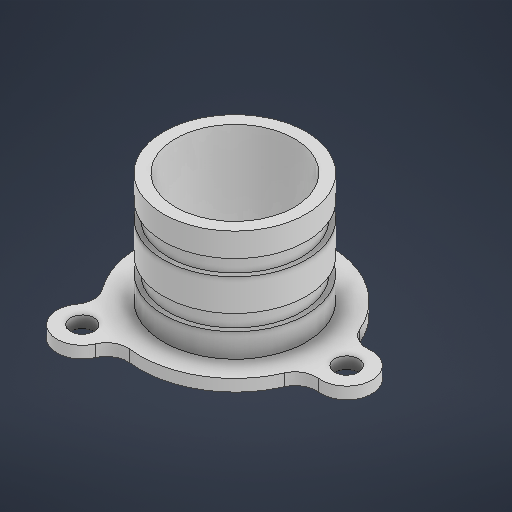
# Autodesk Inventor part: 10
Saved by Autodesk Inventor 2025.4 (Build 294407000, 407)
## iProperties
Created: 2026-05-07
Part Number: 10
Material: Generic
Document SubType Name: Modeling
Designer: VuQuan
Density: 1 g/cm^3
Appearance: Default
Author: VuQuan
Autodesk Inventor part; units mm, degrees
ref_plane "YZ Plane" through (0, 0, 0) normal (1, 0, 0) x (0, 1, 0)
ref_plane "XZ Plane" through (0, 0, 0) normal (0, 1, 0) x (-1, 0, 0)
ref_plane "XY Plane" through (0, 0, 0) normal (0, 0, 1) x (1, 0, 0)
sketch "Sketch1" plane through (0, 0, 0) normal (0, 0, 1) x (1, 0, 0)
  line L0 (0, 0) -> (0, 77.5) construction
  line L1 (45, 77.5) -> (45, 62.5)
  line L2 (45, 62.5) -> (42, 62.5)
  line L3 (42, 62.5) -> (42, 52.5)
  line L4 (42, 52.5) -> (45, 52.5)
  line L5 (45, 52.5) -> (45, 32.5)
  line L6 (45, 32.5) -> (42, 32.5)
  line L7 (42, 32.5) -> (42, 22.5)
  line L8 (42, 22.5) -> (45, 22.5)
  line L9 (45, 22.5) -> (45, 7.5)
  line L10 (45, 77.5) -> (37.5, 77.5)
  line L11 (37.5, 77.5) -> (37.5, 7.5)
  line L12 (37.5, 7.5) -> (45, 7.5)
  dimension "d0" = 3
  dimension "d1" = 15
  dimension "d2" = 10
  dimension "d3" = 20
  dimension "d4" = 7.5
  dimension "d5" = 15
  dimension "d6" = 90
  dimension "d7" = 77.5
  dimension "d8" = 75
  constraints: 26 end point, 8 perpendicular, 3 point on line, 2 collinear, 2 horizontal, 2 vertical
  measures "d0" distance of L7.end L8.end
  measures "d1" distance of L1.start L1.end
  measures "d2" distance of L6.end L7.end
  measures "d3" distance of L4.end L5.end
  measures "d4" vertical distance of L0.start L9.end
  measures "d5" distance of L8.end L9.end
  measures "d6" diameter of L1 L0
  measures "d7" distance from line of L10 L0.start
  measures "d8" diameter of L11 L0
revolve "Revolution1" add sketch "Sketch1" angle 360 about axis through (0, 0, 0) along (0, 1, 0)
sketch "Sketch3" plane through (0, 7.5, 0) normal (0, -1, 0) x (1, 0, 0)
  circle A0 centre (0, 0) radius 45 projected
  circle A1 centre (0, 0) radius 37.5 projected
  circle A2 centre (0, 0) radius 37.5
  circle A3 centre (-35.25, -61.0548) radius 7.5
  circle A4 centre (70.5, 0) radius 7.5
  circle A5 centre (-35.25, 61.0548) radius 7.5
  arc A6 (-20.5753, 67.4308) -> (-48.1091, 51.5341) centre (-35.25, 61.0548) ccw
  arc A7 (-48.1091, 35.6192) -> (-48.1091, -35.6192) centre (0, 0) ccw
  arc A8 (-48.1091, 35.6192) -> (-48.1091, 51.5341) centre (-58.8568, 43.5767) ccw
  arc A9 (-48.1091, -51.5341) -> (-48.1091, -35.6192) centre (-58.8568, -43.5767) ccw
  arc A10 (-48.1091, -51.5341) -> (-20.5753, -67.4308) centre (-35.25, -61.0548) ccw
  arc A11 (-6.7926, -59.4733) -> (-20.5753, -67.4308) centre (-8.3101, -72.7598) ccw
  arc A12 (-6.7926, -59.4733) -> (54.9017, -23.8541) centre (0, 0) ccw
  arc A13 (68.6844, -15.8967) -> (54.9017, -23.8541) centre (67.1669, -29.1831) ccw
  arc A14 (68.6844, -15.8967) -> (68.6844, 15.8967) centre (70.5, 0) ccw
  arc A15 (54.9017, 23.8541) -> (68.6844, 15.8967) centre (67.1669, 29.1831) ccw
  arc A16 (54.9017, 23.8541) -> (-6.7926, 59.4733) centre (0, 0) ccw
  arc A17 (-20.5753, 67.4308) -> (-6.7926, 59.4733) centre (-8.3101, 72.7598) ccw
  point P0 (-20.5753, 67.4308)
  point P1 (-48.1091, -51.5341)
  point P2 (68.6844, -15.8967)
  dimension "d10" = 141
  dimension "d11" = 15
  dimension "d14" = 360
  dimension "d16" = 16
  dimension "d19" = 360
  constraints: 24 point on circle, 16 centre point, 7 coincident, 3 tangent, 1 equal radius, 1 horizontal alignment, 1 vertical alignment, 54 other
  measures "d11" diameter of A3
  measures "d16" radius of A6
extrude "Extrusion1" add sketch "Sketch3" along normal blind 7.5 contours A0 | A17 A16 A15 A14 A13 A12 A11 A10 A9 A7 A8 A6
body "Solid1"
